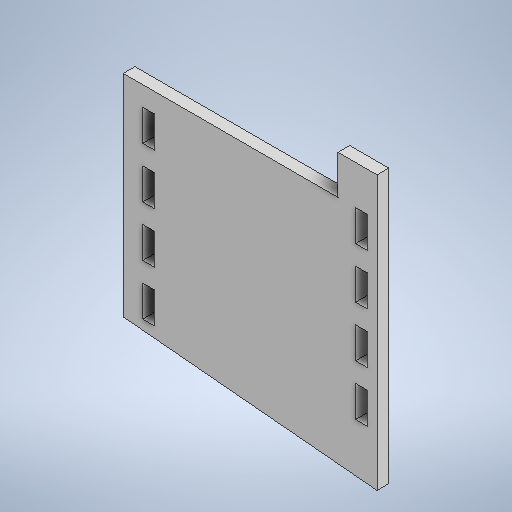
# Autodesk Inventor part: support select pt 1
Saved by Autodesk Inventor 2025.3 (Build 293356000, 356)
## iProperties
Created: 2026-04-27
Part Number: support select pt 1
Material: Generic
Document SubType Name: Modeling
Designer: kamal
Density: 1 g/cm^3
Appearance: Default
Author: kamal
Autodesk Inventor part; units mm, degrees
ref_plane "YZ Plane" through (0, 0, 0) normal (1, 0, 0) x (0, 1, 0)
ref_plane "XZ Plane" through (0, 0, 0) normal (0, 1, 0) x (-1, 0, 0)
ref_plane "XY Plane" through (0, 0, 0) normal (0, 0, 1) x (1, 0, 0)
sketch "Sketch1" plane through (0, 0, 0) normal (0, 0, 1) x (1, 0, 0)
  line L0 (0, 0) -> (0, 54)
  line L1 (0, 54) -> (55, 54)
  line L2 (55, 54) -> (55, 64)
  line L3 (55, 64) -> (65, 64)
  line L4 (65, 64) -> (65, -6)
  line L5 (65, -6) -> (0, 0)
  line L6 (5, 49) -> (8, 49)
  line L7 (8, 49) -> (8, 41)
  line L8 (8, 41) -> (5, 41)
  line L9 (5, 41) -> (5, 49)
  line L10 (5, 36) -> (8, 36)
  line L11 (8, 36) -> (8, 28)
  line L12 (8, 28) -> (5, 28)
  line L13 (5, 28) -> (5, 36)
  line L14 (5, 23) -> (8, 23)
  line L15 (8, 23) -> (8, 15)
  line L16 (8, 15) -> (5, 15)
  line L17 (5, 15) -> (5, 23)
  line L18 (5, 10) -> (8, 10)
  line L19 (8, 10) -> (8, 2)
  line L20 (8, 2) -> (5, 2)
  line L21 (5, 2) -> (5, 10)
  line L22 (59.5, 54) -> (62.5, 54)
  line L23 (62.5, 54) -> (62.5, 46)
  line L24 (62.5, 46) -> (59.5, 46)
  line L25 (59.5, 46) -> (59.5, 54)
  line L26 (59.5, 41) -> (62.5, 41)
  line L27 (62.5, 41) -> (62.5, 33)
  line L28 (62.5, 33) -> (59.5, 33)
  line L29 (59.5, 33) -> (59.5, 41)
  line L30 (59.5, 28) -> (62.5, 28)
  line L31 (62.5, 28) -> (62.5, 20)
  line L32 (62.5, 20) -> (59.5, 20)
  line L33 (59.5, 20) -> (59.5, 28)
  line L34 (59.5, 15) -> (62.5, 15)
  line L35 (62.5, 15) -> (62.5, 7)
  line L36 (62.5, 7) -> (59.5, 7)
  line L37 (59.5, 7) -> (59.5, 15)
  point P0 (6.5, 49)
  point P1 (6.5, 36)
  point P2 (6.5, 23)
  point P3 (6.5, 10)
  point P4 (6.5, 41)
  point P5 (6.5, 28)
  point P6 (6.5, 15)
  point P7 (5, 6)
  point P8 (61, 54)
  point P9 (61, 41)
  point P10 (61, 28)
  point P11 (61, 15)
  point P12 (61, 46)
  point P13 (61, 33)
  point P14 (61, 20)
  point P15 (59.5, 11)
  point P16 (60, 64)
  point P17 (62.5, 37)
  dimension "d0" = 54
  dimension "d1" = 55
  dimension "d2" = 10
  dimension "d3" = 10
  dimension "d4" = 70
  dimension "d5" = 3
  dimension "d6" = 8
  dimension "d7" = 5
  dimension "d8" = 5
  dimension "d9" = 3
  dimension "d10" = 8
  dimension "d11" = 3
  dimension "d12" = 8
  dimension "d13" = 3
  dimension "d14" = 8
  dimension "d15" = 5
  dimension "d16" = 5
  dimension "d17" = 5
  dimension "d18" = 5
  dimension "d19" = 5
  dimension "d20" = 5
  dimension "d21" = 3
  dimension "d22" = 8
  dimension "d23" = 3
  dimension "d24" = 8
  dimension "d25" = 3
  dimension "d26" = 8
  dimension "d27" = 3
  dimension "d28" = 8
  dimension "d29" = 5
  dimension "d30" = 5
  dimension "d31" = 5
  dimension "d32" = 10
  dimension "d33" = 2.5
  dimension "d34" = 2.5
  dimension "d35" = 2.5
  dimension "d36" = 2.5
  constraints: 76 end point, 18 midpoint, 16 parallel, 10 perpendicular, 9 horizontal, 2 vertical
  measures "d0" distance of L0.start L0.end
  measures "d1" distance of L0.end L1.end
  measures "d2" distance of L1.end L2.end
  measures "d3" distance of L2.end L3.end
  measures "d4" distance of L3.end L4.end
  measures "d5" distance of L7.end L8.end
  measures "d6" distance of L6.end L7.end
  measures "d7" distance between parallel lines of L0 L9
  measures "d8" distance from line of L1 point (6.5, 49)
  measures "d9" distance of L11.end L12.end
  measures "d10" distance of L10.end L11.end
  measures "d11" distance of L15.end L16.end
  measures "d12" distance of L14.end L15.end
  measures "d13" distance of L19.end L20.end
  measures "d14" distance of L18.end L19.end
  measures "d15" distance between parallel lines of L0 L13
  measures "d16" distance of point (6.5, 41) point (6.5, 36)
  measures "d17" distance between parallel lines of L0 L17
  measures "d18" distance of point (6.5, 23) point (6.5, 28)
  measures "d19" distance from line of L18 point (6.5, 15)
  measures "d20" distance from line of L0 point (5, 6)
  measures "d21" distance of L23.end L24.end
  measures "d22" distance of L22.end L23.end
  measures "d23" distance of L27.end L29.start
  measures "d24" distance of L27.start L27.end
  measures "d25" distance of L32.start L32.end
  measures "d26" distance of L31.start L32.start
  measures "d27" distance of L35.end L37.start
  measures "d28" distance of L34.end L35.end
  measures "d29" distance of point (61, 46) point (61, 41)
  measures "d30" distance of point (61, 28) point (61, 33)
  measures "d31" distance from line of L34 point (61, 20)
  measures "d32" vertical distance of point (60, 64) point (61, 54)
  measures "d33" distance from line of L4 point (62.5, 37)
  measures "d34" distance between parallel lines of L4 L23
  measures "d35" distance between parallel lines of L4 L31
  measures "d36" distance between parallel lines of L35 L4
extrude "Extrusion1" add sketch "Sketch1" along normal blind 3
body "Solid1"
